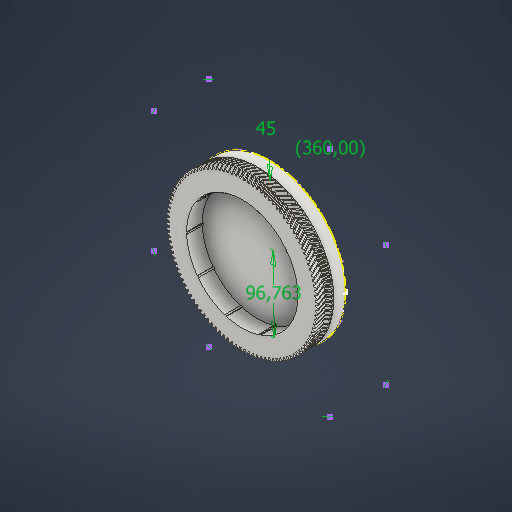
# Autodesk Inventor part: Przekładnia walcowa2
Saved by Autodesk Inventor 2026.1 (Build 301233020, 233B)
## iProperties
CustomPartVersion: 1
Created: 2025-11-16
Part Number: Przekładnia walcowa2
Material: Steel
Document SubType Name: Modeling
Designer: obiwa
Categories: <?xml version="1.0" encoding="UTF-16"?> <MemberInstance><Categories><FamilyTemplate><FamilyTemplateParameter ValueType="xs:double" Id="1" ObjectReferenceKey="da_z" ObjectType="kUserParameterObject"/><FamilyTemplateParameter ValueType="xs:double" Id="2" ObjectReferenceKey="da_b" ObjectType="kUserParameterObject"/><FamilyTemplateParameter ValueType="xs:double" Id="3" ObjectReferenceKey="da_beta" ObjectType="kUserParameterObject"/><FamilyTemplateParameter ValueType="xs:double" Id="4" ObjectReferenceKey="da_da" ObjectType="kUserParameterObject"/><FamilyTemplateParameter ValueType="xs:double" Id="5" ObjectReferenceKey="da_aw" ObjectType="kUserParameterObject"/><FamilyTemplateParameter ValueType="xs:string" Id="6" ObjectReferenceKey="EAIAABAAAACIAQAAAAAAAIAAAAAAAAAA" ObjectType="83910656" SubObjectId="SurfaceGeometry"/></FamilyTemplate><ParamToTemplateMap><ParamToTemplate CategoryParameter="//CategoryParameter[@InternalName='046C89C9-8512-4d59-83FE-43B91F4F132A']" TemplateParameter="1"/><ParamToTemplate CategoryParameter="//CategoryParameter[@InternalName='2552DF32-E462-4b46-AEBF-C6C7768E72AC']" TemplateParameter="2"/><ParamToTemplate CategoryParameter="//CategoryParameter[@InternalName='C9EE641D-15FC-4fae-A226-E94C4372FDD7']" TemplateParameter="3"/><ParamToTemplate><ParamToTemplate CategoryParameter="//CategoryParameter[@InternalName='00B6519A-459B-49c7-AD84-2E56D39A5744']" ConstantValue="0.000000"/></ParamToTemplate><ParamToTemplate><ParamToTemplate CategoryParameter="//CategoryParameter[@InternalName='04B31F0E-C7A6-4894-AA32-9629BEFACF47']" ConstantValue="1.000000"/></ParamToTemplate><ParamToTemplate><ParamToTemplate CategoryParameter="//CategoryParameter[@InternalName='43CBEC2E-7847-49e7-A936-2F7889FCB2D9']" ConstantValue="0.250000"/></ParamToTemplate><ParamToTemplate><ParamToTemplate CategoryParameter="//CategoryParameter[@InternalName='B1EFC894-105D-4ebd-86BF-FA20ED196853']" ConstantValue="0.350000"/></ParamToTemplate><ParamToTemplate><ParamToTemplate CategoryParameter="//CategoryParameter[@InternalName='51175063-3D10-4879-93E8-6246FE8B403D']" ConstantValue="2060000000.000000"/></ParamToTemplate><ParamToTemplate><ParamToTemplate CategoryParameter="//CategoryParameter[@InternalName='A3A52E27-4454-46a9-B0BD-C932399B70AF']" ConstantValue="0.300000"/></ParamToTemplate><ParamToTemplate><ParamToTemplate CategoryParameter="//CategoryParameter[@InternalName='91B76062-C214-41d9-B1B9-14D2AB99603D']" ConstantValue="0.150000"/></ParamToTemplate><ParamToTemplate><ParamToTemplate CategoryParameter="//CategoryParameter[@InternalName='374E806E-8B8A-4dda-A9AA-1039D6500AD2']" ConstantValue="6.666667"/></ParamToTemplate><ParamToTemplate><ParamToTemplate CategoryParameter="//CategoryParameter[@InternalName='2D373A89-B862-43d6-8D0B-0CBF12AB9F6C']" ConstantValue="0.349066"/></ParamToTemplate><ParamToTemplate CategoryParameter="//CategoryParameter[@InternalName='37777632-D6A2-4fac-9D53-DB8ACD95C989']" TemplateParameter="4"/><ParamToTemplate CategoryParameter="//CategoryParameter[@InternalName='FD1017F1-B727-4f7e-9707-0F86F1FF9423']" TemplateParameter="5"/><ParamToTemplate><ParamToTemplate CategoryParameter="//CategoryParameter[@InternalName='9E1B4470-B2D3-4ff1-B813-535BB4CDF51A']" ConstantValue="3520000.000000"/></ParamToTemplate><ParamToTemplate><ParamToTemplate CategoryParameter="//CategoryParameter[@InternalName='F8452263-BFF6-458c-9FB1-07C4B99E95CD']" ConstantValue="11400000.000000"/></ParamToTemplate><ParamToTemplate><ParamToTemplate CategoryParameter="//CategoryParameter[@InternalName='3E3BB259-FD49-497f-8171-6EBC954A3479']" ConstantValue="2.000000"/></ParamToTemplate><ParamToTemplate CategoryParameter="//CategoryParameter[@InternalName='27C3BAF2-7550-4e4b-AE2C-0DB134B7D9B7']" TemplateParameter="6"/></ParamToTemplateMap><Category DisplayName="Gear" InternalName="DC85795E-93AB-48d5-8EEE-5A27447B64BD" Mnemonic="Gear"><CategoryParameter DisplayName="z" InternalName="046C89C9-8512-4d59-83FE-43B91F4F132A" Mnemonic="z"/><CategoryParameter DisplayName="b" InternalName="2552DF32-E462-4b46-AEBF-C6C7768E72AC" Mnemonic="b"/><CategoryParameter DisplayName="||b|" InternalName="C9EE641D-15FC-4fae-A226-E94C4372FDD7" Mnemonic="beta"/><CategoryParameter DisplayName="x" InternalName="00B6519A-459B-49c7-AD84-2E56D39A5744" Mnemonic="x"/><CategoryParameter DisplayName="a*" InternalName="04B31F0E-C7A6-4894-AA32-9629BEFACF47" Mnemonic="a"/><CategoryParameter DisplayName="c*" InternalName="43CBEC2E-7847-49e7-A936-2F7889FCB2D9" Mnemonic="c"/><CategoryParameter DisplayName="r|.f|*" InternalName="B1EFC894-105D-4ebd-86BF-FA20ED196853" Mnemonic="rf"/><CategoryParameter DisplayName="E" InternalName="51175063-3D10-4879-93E8-6246FE8B403D" Mnemonic="E"/><CategoryParameter DisplayName="||m|" InternalName="A3A52E27-4454-46a9-B0BD-C932399B70AF" Mnemonic="mi"/><Category DisplayName="SpurGear" InternalName="26C5A22E-A91E-4dfd-A3B3-23CCAFAE1764" Mnemonic="SpurGear"><CategoryParameter DisplayName="m" InternalName="91B76062-C214-41d9-B1B9-14D2AB99603D" Mnemonic="m"/><CategoryParameter DisplayName="P" InternalName="374E806E-8B8A-4dda-A9AA-1039D6500AD2" Mnemonic="PP"/><CategoryParameter DisplayName="||a|" InternalName="2D373A89-B862-43d6-8D0B-0CBF12AB9F6C" Mnemonic="alpha"/><CategoryParameter DisplayName="d|.a|" InternalName="37777632-D6A2-4fac-9D53-DB8ACD95C989" Mnemonic="da"/><CategoryParameter DisplayName="a|.w|" InternalName="FD1017F1-B727-4f7e-9707-0F86F1FF9423" Mnemonic="aw"/><CategoryParameter DisplayName="||s||.Flim|" InternalName="9E1B4470-B2D3-4ff1-B813-535BB4CDF51A" Mnemonic="sFlim"/><CategoryParameter DisplayName="||s||.Hlim|" InternalName="F8452263-BFF6-458c-9FB1-07C4B99E95CD" Mnemonic="sHlim"/><CategoryParameter DisplayName="typ" InternalName="3E3BB259-FD49-497f-8171-6EBC954A3479" Mnemonic="type"/><CategoryParameter DisplayName="PitchDiameter" InternalName="27C3BAF2-7550-4e4b-AE2C-0DB134B7D9B7" Mnemonic="IDS_PITCHDIAM"/></Category></Category></Categories></MemberInstance>
Density: 1 g/cm^3
Appearance: Steel
Author: obiwa
Autodesk Inventor part; units mm, degrees
sketch "Sketch1" plane through (0, 0, 0) normal (0, 0, 1) x (1, 0, 0)
  circle A0 centre (0, 0) radius 96.7628
  dimension "d0" = 193.5256
  constraints: 1 centre point
  measures "d0" diameter of A0
extrude "Extrusion1" add sketch "Sketch1" along normal blind 10
ref_plane "Work Plane2" through (0, 0, 5) normal (0, 0, 1) x (1, 0, 0)
sketch "Sketch2" plane through (0, 0, 0) normal (0, 0, -1) x (-1, 0, 0)
  circle A0 centre (0, 0) radius 96.7628 projected
  circle A1 centre (0, 0) radius 95.2628
  dimension "d3" = 190.5256
  constraints: 1 centre point, 1 coincident
  measures "d3" diameter of A1
surface extrude "Średnica podziałowa" sketch "Sketch2" against normal through all shown no curves A1
ref_plane "Work Plane8" through (0, 0, 0) normal (0.9995922, 0.0285561, 0) x (0, 0, 1)
ref_plane "Work Plane9" through (0, 0, 0) normal (1, 0, 0) x (0, 1, 0)
spur gear teeth "Przekładnia walcowa" teeth 110 pitch diameter 190.5256 tip diameter 193.5256 root diameter 186.7756 face width 10 helix angle 30 hand right start plane through (0, 0, 0) normal (0, 0, -1) x (-1, 0, 0)
mirror "Odbij1" about plane through (0, 0, 10) normal (0, 0, 1)
sketch "Szkic3" plane through (0, 0, 20) normal (0, 0, 1) x (-0.2542183, 0.9671469, 0)
  circle A0 centre (0, 0) radius 71
  dimension "d49" = 142
  constraints: 1 centre point, 1 coincident
  measures "d49" diameter of A0
extrude "Wyciągnięcie proste2" cut sketch "Szkic3" against normal through all
sketch "Szkic4" plane through (0, 0, 0) normal (0, 0, -1) x (-1, 0, 0)
  circle A0 centre (0, 0) radius 71 projected
  line L0 (71, 0) -> (70, 0)
  line L1 (70, 0) -> (70, -2)
  line L2 (70, -2) -> (71, -2)
  line L3 (71, -2) -> (71, 0)
  line L4 (56.6312, 41.145) -> (57.8068, 39.5269)
  line L5 (57.8068, 39.5269) -> (58.6158, 40.1147)
  line L6 (58.6158, 40.1147) -> (57.4402, 41.7328)
  line L7 (57.4402, 41.7328) -> (56.6312, 41.145)
  line L8 (21.6312, 66.574) -> (23.5333, 65.9559)
  line L9 (23.5333, 65.9559) -> (23.8423, 66.907)
  line L10 (23.8423, 66.907) -> (21.9402, 67.525)
  line L11 (21.9402, 67.525) -> (21.6312, 66.574)
  line L12 (-21.6312, 66.574) -> (-19.7291, 67.192)
  line L13 (-19.7291, 67.192) -> (-20.0381, 68.143)
  line L14 (-20.0381, 68.143) -> (-21.9402, 67.525)
  line L15 (-21.9402, 67.525) -> (-21.6312, 66.574)
  line L16 (-56.6312, 41.145) -> (-55.4556, 42.763)
  line L17 (-55.4556, 42.763) -> (-56.2646, 43.3508)
  line L18 (-56.2646, 43.3508) -> (-57.4402, 41.7328)
  line L19 (-57.4402, 41.7328) -> (-56.6312, 41.145)
  line L20 (-70, 0) -> (-70, 2)
  line L21 (-70, 2) -> (-71, 2)
  line L22 (-71, 2) -> (-71, 0)
  line L23 (-71, 0) -> (-70, 0)
  line L24 (-56.6312, -41.145) -> (-57.8068, -39.5269)
  line L25 (-57.8068, -39.5269) -> (-58.6158, -40.1147)
  line L26 (-58.6158, -40.1147) -> (-57.4402, -41.7328)
  line L27 (-57.4402, -41.7328) -> (-56.6312, -41.145)
  line L28 (-21.6312, -66.574) -> (-23.5333, -65.9559)
  line L29 (-23.5333, -65.9559) -> (-23.8423, -66.907)
  line L30 (-23.8423, -66.907) -> (-21.9402, -67.525)
  line L31 (-21.9402, -67.525) -> (-21.6312, -66.574)
  line L32 (21.6312, -66.574) -> (19.7291, -67.192)
  line L33 (19.7291, -67.192) -> (20.0381, -68.143)
  line L34 (20.0381, -68.143) -> (21.9402, -67.525)
  line L35 (21.9402, -67.525) -> (21.6312, -66.574)
  line L36 (56.6312, -41.145) -> (55.4556, -42.763)
  line L37 (55.4556, -42.763) -> (56.2646, -43.3508)
  line L38 (56.2646, -43.3508) -> (57.4402, -41.7328)
  line L39 (57.4402, -41.7328) -> (56.6312, -41.145)
  point P0 (-70.9718, 2)
  point P1 (-71, 0)
  point P2 (56.2418, -43.3342)
  point P3 (70.9718, -2)
  point P4 (-56.2418, 43.3342)
  point P5 (-20.0294, 68.1163)
  point P6 (23.8336, 66.8802)
  point P7 (58.593, 40.0982)
  point P8 (-58.593, -40.0982)
  point P9 (-23.8336, -66.8802)
  point P10 (20.0294, -68.1163)
  dimension "d86" = 1
  dimension "d87" = 2
  dimension "d90" = 360
  constraints: 80 end point, 2 parallel, 1 horizontal, 1 perpendicular, 83 other
  measures "d86" distance of L2.end L1.end
  measures "d87" distance of L1.end L0.end
sketch "Szkic6" plane through (0, 0, 0) normal (0, 0, -1) x (-1, 0, 0)
  arc A0 (26.5976, -93.0355) -> (27.9234, -92.6462) centre (0, 0) ccw projected
  circle A1 centre (0, 0) radius 96.7628
  point P0 (27.9234, -92.6462)
  constraints: 1 coincident, 3 other
extrude "Wyciągnięcie proste3" add sketch "Szkic6" along normal blind 15 separate body
sketch "Szkic7" plane through (0, 0, -15) normal (0, 0, -1) x (-1, 0, 0)
  circle A0 centre (0, 0) radius 96.7628 projected
  arc A1 (-57.4332, -77.8747) -> (-56.3154, -78.6868) centre (0, 0) ccw projected
  circle A2 centre (0, 96.7628) radius 22.5
  arc A3 (-41.9992, 87.1728) -> (-17.7524, 110.5868) centre (-77.3804, 148.0743) ccw
  line L0 (0, 96.7628) -> (0, 0)
  arc A4 (17.7524, 110.5868) -> (41.9992, 87.1728) centre (77.3804, 148.0743) ccw
  arc A5 (-87.1728, -41.9992) -> (-110.5868, -17.7524) centre (-148.0743, -77.3804) ccw
  circle A6 centre (-96.7628, 0) radius 22.5
  arc A7 (-110.5868, 17.7524) -> (-87.1728, 41.9992) centre (-148.0743, 77.3804) ccw
  arc A8 (41.9992, -87.1728) -> (17.7524, -110.5868) centre (77.3804, -148.0743) ccw
  circle A9 centre (0, -96.7628) radius 22.5
  arc A10 (-17.7524, -110.5868) -> (-41.9992, -87.1728) centre (-77.3804, -148.0743) ccw
  arc A11 (87.1728, 41.9992) -> (110.5868, 17.7524) centre (148.0743, 77.3804) ccw
  circle A12 centre (96.7628, 0) radius 22.5
  arc A13 (110.5868, -17.7524) -> (87.1728, -41.9992) centre (148.0743, -77.3804) ccw
  point P0 (-1.3309, -96.7538)
  point P1 (17.7524, 110.5868)
  point P2 (41.9992, 87.1728)
  point P3 (110.5868, -17.7524)
  point P4 (87.1728, 41.9992)
  point P5 (87.1728, -41.9992)
  point P6 (-17.7524, -110.5868)
  point P7 (41.9992, -87.1728)
  point P8 (-41.9992, -87.1728)
  point P9 (-110.5868, 17.7524)
  point P10 (-87.1728, -41.9992)
  point P11 (-87.1728, 41.9992)
  dimension "d75" = 45
  dimension "d54" = 96.763
  dimension "d82" = 360
  constraints: 18 point on circle, 8 centre point, 3 symmetric about line, 2 end point, 1 vertical, 54 other
  measures "d54" distance of A0.centre point (-1.331, -96.754)
extrude "Wyciągnięcie proste10" add sketch "Szkic4" against normal blind 20 contours A0 L2 L1 L0 | L5 L4 L7 A0 | L38 L37 A0 | A0 L37 L36 L39 | L9 L8 L11 A0 | A0 L33 L32 L35 | L13 L12 L15 A0 | A0 L29 L28 L31 | L17 L16 L19 A0 | A0 L25 L24 L27 | L21 L20 L23 A0 bodies 1
equation "\"d0\" = da_da"
equation "\"d1\" = da_b"
equation "\"d3\" = da_d"
equation "\"d16\" = da_aw"
equation "\"d43\" = da_aw"
equation "\"d46\" = da_aw"
equation "\"da_da\" = 193.525589"
equation "\"da_b\" = 10"
equation "\"da_d\" = 190.525589"
equation "\"da_aw\" = 112.583302"
body "Solid1"
body "Srf1"
